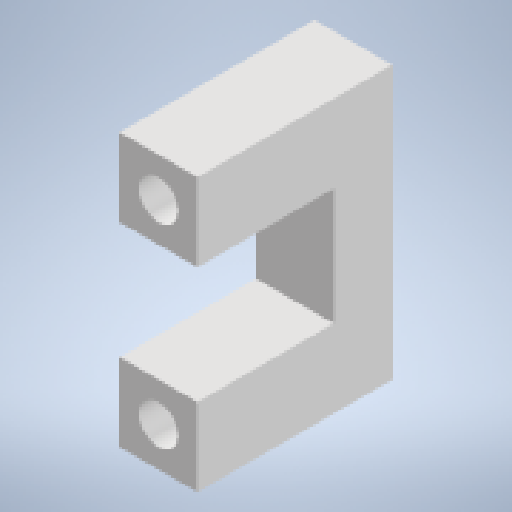
# Autodesk Inventor part: крепление для крепления ремня
Saved by Autodesk Inventor 2024.2 (Build 282272000, 272)
## iProperties
Created: 2026-02-02
Part Number: крепление для крепления ремня
Material: Типовые
Document SubType Name: Modeling
Designer: Service
Density: 1 g/cm^3
Appearance: По умолчанию
Author: Service
Autodesk Inventor part; units mm, degrees
ref_plane "YZ Plane" through (0, 0, 0) normal (1, 0, 0) x (0, 1, 0)
ref_plane "XZ Plane" through (0, 0, 0) normal (0, 1, 0) x (-1, 0, 0)
ref_plane "XY Plane" through (0, 0, 0) normal (0, 0, 1) x (1, 0, 0)
sketch "Эскиз1" plane through (0, 0, 0) normal (0, 0, 1) x (1, 0, 0)
  circle A0 centre (-18.4646, -5) radius 1
  circle A1 centre (-18.4646, 5) radius 1
  circle A2 centre (21.5354, 0) radius 2.5
  circle A3 centre (-18.4646, -25) radius 2.5
  circle A4 centre (-18.4646, 25) radius 2.5
  line L0 (-30, 30) -> (30, 30)
  line L1 (30, 30) -> (30, -30)
  line L2 (30, -30) -> (-30, -30)
  line L3 (-30, -30) -> (-30, 30)
  line L4 (-20.4646, 7) -> (-16.4646, 7)
  line L5 (-16.4646, 7) -> (-16.4646, 3)
  line L6 (-16.4646, 3) -> (-20.4646, 3)
  line L7 (-20.4646, 3) -> (-20.4646, 7)
  line L8 (-20.4646, -3) -> (-16.4646, -3)
  line L9 (-16.4646, -3) -> (-16.4646, -7)
  line L10 (-16.4646, -7) -> (-20.4646, -7)
  line L11 (-20.4646, -7) -> (-20.4646, -3)
  point P0 (0, 0)
  point P1 (-18.4646, -7)
  dimension "d1" = 2
  dimension "d2" = 2
  dimension "d3" = 2
  dimension "d4" = 2
  dimension "d5" = 2
  dimension "d6" = 2
  dimension "d7" = 2
  constraints: 24 end point, 5 centre point, 4 horizontal, 4 parallel, 2 perpendicular, 2 vertical, 1 midpoint, 1 point on line, 14 other
  measures "d1" distance from line of L10 A0.centre
  measures "d2" distance from line of L11 A0.centre
  measures "d3" distance from line of L8 A0.centre
  measures "d4" distance from line of A0.centre L9
  measures "d5" distance from line of L6 A1.centre
  measures "d6" distance from line of L5 A1.centre
  measures "d7" distance from line of L4 A1.centre
extrude "Выдавливание1" add sketch "Эскиз1" against normal blind 10 contours L4 L5 L6 L7 | L8 L9 L10 L11
sketch "Эскиз2" plane through (0, 0, -10) normal (0, 0, -1) x (-1, 0, 0)
  line L0 (16.4646, 3) -> (20.4646, 3)
  line L1 (20.4646, 3) -> (20.4646, -3)
  line L2 (20.4646, -3) -> (16.4646, -3)
  line L3 (16.4646, -3) -> (16.4646, 3)
  line L4 (16.4646, 3) -> (20.4646, 3) projected
  line L5 (16.4646, 7) -> (16.4646, 3) projected
  point P0 (0, 0)
  constraints: 8 end point, 2 collinear, 2 parallel, 1 horizontal, 1 perpendicular
extrude "Выдавливание2" add sketch "Эскиз2" against normal blind 3
